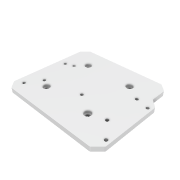
# Autodesk Inventor part: PWTR-0131
Saved by Autodesk Inventor 2021.1 (Build 251245000, 245)
## iProperties
Created: 2020-09-03
Part Number: PWTR-0131
Material: Aluminum 6061
Document SubType Name: Modeling
Designer: alid
Density: 2.7 g/cm^3
Appearance: Aluminum - Flat
Description: Engine Mount Adapter Plate
Mass: 1185.04 g
Surface Area: 997.593 cm^2
Volume: 438.902 cm^3
Author: alid
Revision Number: A
Autodesk Inventor part; units mm, degrees
ref_plane "YZ Plane" through (0, 0, 0) normal (1, 0, 0) x (0, 1, 0)
ref_plane "XZ Plane" through (0, 0, 0) normal (0, 1, 0) x (-1, 0, 0)
ref_plane "XY Plane" through (0, 0, 0) normal (0, 0, 1) x (1, 0, 0)
sketch "Sketch1" plane through (0, 0, 0) normal (0, 0, 1) x (1, 0, 0)
  line L0 (-100, -120) -> (100, -120)
  line L1 (100, -120) -> (100, 120)
  line L2 (100, 120) -> (-100, 120)
  line L3 (-100, 120) -> (-100, -120)
  line L4 (-100, -120) -> (100, 120) construction
  line L5 (100, -120) -> (-100, 120) construction
  circle A0 centre (0, 0) radius 75 construction
  line L6 (0, 0) -> (0, 75)
  line L7 (0, 0) -> (-53.033, 53.033) construction
  line L8 (50, -120) -> (50, -105)
  line L9 (50, -105) -> (100, -105)
  dimension "d0" = 200
  dimension "d1" = 240
  dimension "d7" = 150
  dimension "d8" = 45
  dimension "d50" = 15
  dimension "d51" = 50
  constraints: 20 end point, 2 midpoint, 2 parallel, 2 perpendicular, 2 point on circle, 2 point on line, 2 vertical, 1 centre point, 1 coincident, 1 horizontal
  measures "d0" distance of L2.end L1.end
  measures "d1" distance of L1.end L0.end
  measures "d7" diameter of A0
  measures "d8" angle of L6 L7
  measures "d50" distance of L8.start L8.end
  measures "d51" distance of L8.end L9.end
extrude "Extrusion1" add sketch "Sketch1" against normal blind 10
hole "Hole1" at (-53.033, 53.033, 0) direction (0, 0, -1) diameter 9 end through all counterbore diameter 15 counterbore depth 5 clearance for "Socket Head Cap Screw ISO 4762" size "M8" standard "ISO"
pattern_circular "Circular Pattern1" count 4 over 360 about axis through (0, 0, -10) along (0, 0, 1) of "Hole1"
sketch "Sketch2" plane through (0, 0, 0) normal (0, 0, 1) x (1, 0, 0)
  line L0 (-75, -112) -> (25, -112)
  line L1 (25, -112) -> (25, 92)
  line L2 (25, 92) -> (-75, 92)
  line L3 (-75, 92) -> (-75, -112)
  line L4 (-75, -112) -> (25, 92) construction
  line L5 (25, -112) -> (-75, 92) construction
  point P0 (0, 0)
  point P1 (-25, -10)
  dimension "d19" = 100
  dimension "d20" = 204
  dimension "d42" = 10
  dimension "d43" = 25
  constraints: 12 end point, 3 coincident, 2 midpoint, 2 parallel, 1 horizontal, 1 perpendicular
  measures "d19" distance of L2.end L1.end
  measures "d20" distance of L1.end L0.end
  measures "d42" vertical distance of point (-25, -10) point (0, 0)
  measures "d43" horizontal distance of point (0, 0) point (-25, -10)
hole "Hole2" at (25, -112, 0) direction (0, 0, -1) diameter 6.647 end through all thread size "M8x1.25" class "6H" standard "ISO Metric profile"
pattern_sketch "GX100" of "Hole2" from (25, -112, 0) copies at (-75, -112, 0) at (25, 92, 0) at (-75, 92, 0) at (-25, -10, 0)
sketch "Sketch3" plane through (0, 0, 0) normal (0, 0, 1) x (1, 0, 0)
  line L0 (-43.075, -85.174) -> (31.925, -85.174)
  line L1 (31.925, -85.174) -> (31.925, 72.826)
  line L2 (31.925, 72.826) -> (-43.075, 72.826)
  line L3 (-43.075, 72.826) -> (-43.075, -85.174)
  line L4 (-43.075, -85.174) -> (31.925, 72.826) construction
  line L5 (31.925, -85.174) -> (-43.075, 72.826) construction
  point P0 (0, 0)
  point P1 (-5.575, -6.174)
  dimension "d32" = 75
  dimension "d33" = 158
  dimension "d45" = 6.174
  dimension "d46" = 5.575
  constraints: 12 end point, 3 coincident, 2 midpoint, 2 parallel, 1 horizontal, 1 perpendicular
  measures "d32" distance of L2.end L1.end
  measures "d33" distance of L1.end L0.end
  measures "d45" vertical distance of point (0, 0) point (-5.575, -6.174)
  measures "d46" horizontal distance of point (0, 0) point (-5.575, -6.174)
hole "Hole3" at (-43.075, 72.826, 0) direction (0, 0, -1) diameter 6.647 end through all thread size "M8x1.25" class "6H" standard "ISO Metric profile"
pattern_sketch "GX150" of "Hole3" from (-43.075, 72.826, 0) copies at (-43.075, -85.174, 0) at (31.925, -85.174, 0) at (31.925, 72.826, 0)
move faces "Move1" translate (0, -10, 0) faces at (33.3333, 120, -3.3333)
extrude "Extrusion2" cut sketch "Sketch1" against normal through all contours L8 L9 L1 L0
chamfer "Chamfer2" distance 15 angle 45 5 edges at (100, -105, -5) (-100, -120, -5) (-100, 110, -5) (100, 110, -5) (50, -120, -5)
fillet "Fillet2" radius 5 13 edges at (-85.0001, -120, -5) (35.0001, -120, -5) (50, -105.0001, 0) (50, -105.0001, -5) (50, -105.0001, -10) (50, -105, -5) (85.0001, -105, -5) (100, -90.0001, -5) (100, 95.0001, -5) (85.0001, 110, -5) (-100, -105.0001, -5) (-100, 95.0001, -5) (-85.0001, 110, -5)
body "Solid1"
